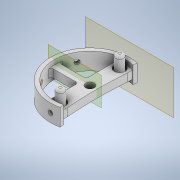
# Autodesk Inventor part: Verbindungsring_2_3
Saved by Autodesk Inventor 2020 (Build 240168000, 168)
## iProperties
Created: 2022-02-05
Part Number: Verbindungsring_2_3
Material: Generisch
Document SubType Name: Modeling
Designer: sp
Density: 1 g/cm^3
Appearance: Vorgabe
Author: sp
## iProperties of the stored document _3D-Druck.ipt
Created: 2022-05-01
Part Number: _3D-Druck
Material: Generisch
Document SubType Name: Modeling
Designer: sp
Density: 1 g/cm^3
Appearance: Vorgabe
Author: sp
Autodesk Inventor part; units mm, degrees
ref_plane "YZ Plane" through (0, 0, 0) normal (1, 0, 0) x (0, 1, 0)
ref_plane "XZ Plane" through (0, 0, 0) normal (0, 1, 0) x (-1, 0, 0)
sketch "Skizze5" plane through (0, 0, 0) normal (0, 1, 0) x (-1, 0, 0)
  circle A0 centre (0, 0) radius 27
  circle A1 centre (0, 0) radius 30
  dimension "d23" = 60
  dimension "d24" = 54
  constraints: 2 centre point, 2 coincident
  measures "d23" diameter of A1
  measures "d24" diameter of A0
extrude "Extrusion4" add sketch "Skizze5" along normal mid plane 2
sketch "Skizze6" plane through (0, 0, 0) normal (0, 1, 0) x (-1, 0, 0)
  circle A0 centre (0, 0) radius 27
  circle A1 centre (0, 0) radius 30
  dimension "d27" = 54
  dimension "d28" = 60
  constraints: 2 centre point, 2 coincident
  measures "d27" diameter of A0
  measures "d28" diameter of A1
extrude "Extrusion5" add sketch "Skizze6" along normal mid plane 13
ref_plane "Arbeitsebene5" through (0, 0, -30) normal (0, 0, 1) x (1, 0, 0)
sketch "Skizze7" plane through (0, 0, -30) normal (0, 0, 1) x (1, 0, 0)
  circle A0 centre (0, 0) radius 1.75
  line L0 (-34.5015, 0) -> (40.4508, 0) construction
  dimension "d33" = 3.5
  constraints: 2 end point, 1 centre point, 1 coincident, 1 horizontal, 1 point on line
  measures "d33" diameter of A0
extrude "Extrusion6" cut sketch "Skizze7" along normal blind 5
pattern_circular "Runde Anordnung2" count 3 over 360 about axis through (0, -10, 0) along (0, 1, 0) of "Extrusion6"
sketch "Skizze8" plane through (0, 0, 0) normal (0, 1, 0) x (-1, 0, 0)
  line L0 (-16.7844, 0) -> (18.1163, 0) construction
  line L1 (0, -12.3348) -> (0, 12.3348) construction
  circle A0 centre (0, -22.5) radius 1.75
  circle A1 centre (0, 22.5) radius 1.75
  circle A2 centre (0, -22.5) radius 5
  circle A3 centre (0, 22.5) radius 5
  line L2 (-5, -22.5) -> (5, -22.5)
  line L3 (5, -22.5) -> (5, 22.5)
  line L4 (5, 22.5) -> (-5, 22.5)
  line L5 (-5, 22.5) -> (-5, -22.5)
  circle A4 centre (0, 0) radius 27.0734
  line L6 (-29, -3) -> (29, -3)
  line L7 (29, -3) -> (29, 3)
  line L8 (29, 3) -> (-29, 3)
  line L9 (-29, 3) -> (-29, -3)
  line L10 (6, -28.2976) -> (-6, -28.2976)
  line L11 (-6, -28.2976) -> (-6, 28.5157)
  line L12 (-6, 28.5157) -> (6, 28.5157)
  line L13 (6, 28.5157) -> (6, -28.2976)
  point P0 (5, -3)
  point P1 (26.9066, -3)
  point P2 (26.9066, 3)
  point P3 (5, 3)
  point P4 (2.215, 26.9826)
  point P5 (-2.215, 26.9826)
  point P6 (-5, 3)
  point P7 (-26.9066, 3)
  point P8 (-26.9066, -3)
  point P9 (-5, -3)
  point P10 (-2.215, -26.9826)
  point P11 (2.215, -26.9826)
  point P12 (6, -3)
  point P13 (-6, -3)
  point P14 (-6, 3)
  point P15 (6, 3)
  dimension "d43" = 10
  dimension "d44" = 10
  dimension "d40" = 3.5
  dimension "d41" = 3.5
  dimension "d42" = 45
  dimension "d45" = 6
  dimension "d46" = 58
  dimension "d70" = 12
  constraints: 28 end point, 6 parallel, 4 horizontal, 3 centre point, 3 coincident, 3 perpendicular, 3 point on line, 1 midpoint, 1 symmetric about line, 1 vertical, 9 other
  measures "d40" diameter of A0
  measures "d41" diameter of A1
  measures "d42" distance of A1.centre A0.centre
  measures "d45" distance of L6.end L7.end
  measures "d46" distance of L7.end L8.end
  measures "d70" distance between parallel lines of L11 L13
extrude "Extrusion7" add sketch "Skizze8" along normal mid plane 6 contours L2 A0 | L2 A2 A4 A0 | A0 L2 A2 | A0 L2 | L3 L6 L13 A4 A2 | A2 L5 L6 L3 | A2 A4 L11 L6 L5 | A4 L13 L10 L11 A2 | A2 A4 | L6 L5 L8 L3 | L3 L8 L13 L6 | L6 L11 L8 L5 | L8 L5 A3 L3 | L3 A3 A4 L13 L8 | L13 L8 A4 L6 | L8 L11 A4 A3 L5 | L6 A4 L8 L11 | L4 A1 A3 A4 | A3 L4 A1 | A4 A3 | A3 A4 L11 L12 L13 | L4 A1 | A1 L4
sketch "Skizze10" plane through (0, 3, 0) normal (0, 1, 0) x (1, 0, 0)
  circle A0 centre (0, 0) radius 3.25
  dimension "d55" = 6.5
  constraints: 1 centre point, 1 coincident
  measures "d55" diameter of A0
extrude "Extrusion9" cut sketch "Skizze10" against normal through all
sketch "Skizze11" plane through (0, 0, 0) normal (0, 1, 0) x (-1, 0, 0)
  circle A0 centre (0, 0) radius 30 projected
  arc A1 (-6.6356, -29.2569) -> (-6.5303, 29.2806) centre (-293.6866, 0.5285) ccw
  line L0 (-6.5303, -28.2237) -> (-6.5303, 29.2806) construction
  line L1 (-6.5303, -28.2237) -> (50.9741, -28.2237) construction
  circle A2 centre (0, 0) radius 30
  point P0 (-6.6356, -29.2569)
  dimension "d58" = 90
  constraints: 4 end point, 3 point on circle, 1 centre point, 1 coincident, 1 horizontal, 1 perpendicular, 5 other
  measures "d58" angle of L1 L0
extrude "Extrusion10" cut sketch "Skizze11" along normal mid plane 35 contours A1 A0 picked at (-13.4295, 1.248)
mirror "Spiegeln2" about plane through (0, 0, 0) normal (0, 0, 1) of "Extrusion6", "Runde Anordnung2"
sketch "Skizze12" plane through (0, 3, 0) normal (0, 1, 0) x (1, 0, 0)
  circle A0 centre (0, 22.5) radius 1.75 projected
  circle A1 centre (0, 22.5) radius 3
  circle A2 centre (0, -22.5) radius 1.75 projected
  circle A3 centre (0, -22.5) radius 3
  point P0 (0, 0)
  dimension "d63" = 6
  dimension "d64" = 6
  constraints: 2 centre point, 2 coincident
  measures "d63" diameter of A1
  measures "d64" diameter of A3
extrude "Extrusion11" add sketch "Skizze12" along normal blind 10 contours A0 | A1 | A2 | A3
fillet "Rundung7" radius 2 2 edges at (-3, 13, -22.5) (-3, 13, 22.5)
fillet "Rundung8" radius 2 2 edges at (-6, 0, -3) (-6, 0, 3)
fillet "Rundung9" radius 2 2 edges at (-26.8328, 0, -3) (-26.8328, 0, 3)
sketch "Skizze14" plane through (0, 3, 0) normal (0, 1, 0) x (1, 0, 0)
  circle A0 centre (0, -22.5) radius 1 projected
  circle A1 centre (0, -22.5) radius 3
  circle A2 centre (0, 22.5) radius 1 projected
  circle A3 centre (0, 22.5) radius 3
  circle A4 centre (0, 22.5) radius 3 projected
  circle A5 centre (0, 22.5) radius 4.1
  circle A6 centre (0, -22.5) radius 4.1
  point P0 (0, 0)
  dimension "d73" = 8.2
  dimension "d74" = 8.2
  constraints: 4 centre point, 4 coincident
  measures "d73" diameter of A5
  measures "d74" diameter of A6
extrude "Extrusion13" cut sketch "Skizze14" against normal blind 2 contours A5 | A6
ref_plane "Arbeitsebene6" through (0, 0, 0) normal (0, 0, 1) x (1, 0, 0)
